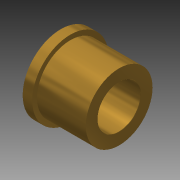
# Autodesk Inventor part: Ball Shisting Shaft Outline Sketch
Saved by Autodesk Inventor 2013 (Build 170138000, 138)
## iProperties
Created: 2013-06-04
Part Number: Ball Shisting Shaft Outline Sketch
Material: Generic
Document SubType Name: Modeling
Designer: mvarma
Density: 1 g/cm^3
Author: mvarma
Autodesk Inventor part; units mm, degrees
ref_plane "YZ Plane" through (0, 0, 0) normal (1, 0, 0) x (0, 1, 0)
ref_plane "XZ Plane" through (0, 0, 0) normal (0, 1, 0) x (-1, 0, 0)
ref_plane "XY Plane" through (0, 0, 0) normal (0, 0, 1) x (1, 0, 0)
sketch "Sketch1" plane through (0, 0, 0) normal (0, 0, 1) x (1, 0, 0)
  line L0 (0, 0) -> (0, 5.5563) construction
  line L1 (0, 0) -> (7.1437, 0) construction
  line L2 (7.1437, 0) -> (7.3977, 0) construction
  line L3 (0, 6.35) -> (7.1437, 6.35) construction
  line L4 (7.1437, 6.35) -> (7.1437, 0) construction
  line L5 (0, 5.5563) -> (7.1437, 5.5563)
  line L6 (7.1437, 6.35) -> (7.1437, 7.9375) construction
  line L7 (7.1437, 7.9375) -> (33.4328, 7.9375) construction
  line L8 (33.4328, 0) -> (33.4328, 7.9375) construction
  line L9 (33.4328, 7.3323) -> (36.6078, 7.3323) construction
  line L10 (36.6078, 7.3323) -> (36.6078, 0) construction
  line L11 (36.6078, 0) -> (33.4328, 0) construction
  line L12 (36.6078, 6.35) -> (44.0055, 6.35) construction
  line L13 (44.0055, 6.35) -> (44.0055, 0) construction
  line L14 (36.6078, 0) -> (36.8618, 0) construction
  line L15 (36.8618, 0) -> (44.0055, 0) construction
  line L16 (36.8618, 0) -> (36.8618, 6.35) construction
  line L17 (7.1437, 5.5563) -> (8.1153, 5.5563)
  line L18 (16.4059, 7.874) -> (17.6759, 7.874) construction
  line L19 (0, 3.1115) -> (44.0055, 3.1115) construction
  line L20 (0, 5.1753) -> (44.0055, 5.1753) construction
  line L21 (7.3977, 0) -> (7.3977, 7.9375) construction
  line L22 (7.3977, 0) -> (8.1915, 0) construction
  line L23 (8.1915, 0) -> (8.1915, 7.9375) construction
  line L24 (8.1915, 7.9375) -> (8.1915, 25.0214) construction
  line L25 (8.1915, 25.0214) -> (12.954, 25.0214) construction
  line L26 (12.954, 25.0214) -> (12.954, 0) construction
  line L27 (12.954, 0) -> (8.1915, 0) construction
  line L28 (12.954, 17.4625) -> (20.2882, 17.4625) construction
  line L29 (12.954, 25.0214) -> (17.7165, 25.0214) construction
  line L30 (17.7165, 25.0214) -> (17.7165, 0) construction
  line L31 (17.7165, 0) -> (12.954, 0) construction
  line L32 (20.2882, 17.4625) -> (20.2882, 0) construction
  line L33 (20.2882, 0) -> (17.7165, 0) construction
  line L34 (20.2882, 0) -> (21.082, 0) construction
  line L35 (21.082, 0) -> (21.082, 14.2875) construction
  line L36 (21.082, 14.2875) -> (20.2882, 14.2875) construction
  line L37 (7.3977, 7.9375) -> (7.3977, 14.2875) construction
  line L38 (7.3977, 14.2875) -> (8.1915, 14.2875) construction
  line L39 (21.082, 30.0415) -> (25.8445, 30.0415) construction
  line L40 (25.8445, 30.0415) -> (25.8445, 0) construction
  line L41 (25.8445, 0) -> (21.082, 0) construction
  line L42 (25.8445, 30.0415) -> (30.607, 30.0415) construction
  line L43 (30.607, 30.0415) -> (30.607, 0) construction
  line L44 (25.8445, 0) -> (30.607, 0) construction
  line L45 (25.8445, 17.4625) -> (33.1787, 17.4625) construction
  line L46 (33.1787, 17.4625) -> (33.1787, 0) construction
  line L47 (33.1787, 0) -> (30.607, 0) construction
  line L48 (21.082, 14.2875) -> (21.082, 30.0415) construction
  line L49 (33.1787, 0) -> (33.4328, 0) construction
  line L50 (10.5727, 25.0214) -> (10.5727, 0) construction
  line L51 (23.4632, 30.0415) -> (23.4632, 0) construction
  circle A0 centre (10.5727, 7.5565) radius 2.3813 construction
  circle A1 centre (10.5727, 5.4928) radius 2.3813 construction
  line L52 (8.9893, 7.874) -> (10.2593, 7.874) construction
  circle A2 centre (23.4632, 5.4928) radius 2.3812 construction
  circle A3 centre (23.4632, 7.5565) radius 2.3812 construction
  line L53 (23.0177, 7.874) -> (24.0459, 7.874) construction
  line L54 (13.843, 5.1752) -> (11.7793, 3.1115) construction
  line L55 (20.193, 5.1752) -> (22.2567, 3.1115) construction
  line L56 (9.9377, 5.1753) -> (7.874, 3.1115) construction
  line L57 (9.6837, 5.1752) -> (8.1153, 3.6068) construction
  line L58 (0, 3.5719) -> (8.0804, 3.5719)
  line L59 (0, 3.5719) -> (-1.5875, 3.5719)
  line L60 (-1.5875, 3.5719) -> (-1.5875, 6.35)
  line L61 (-1.5875, 6.35) -> (0, 6.35)
  line L62 (25.9207, 7.9375) -> (25.9207, 0) construction
  line L63 (24.0982, 5.1752) -> (26.162, 3.1115) construction
  line L64 (25.9207, 5.5563) -> (27.3897, 3.1115) construction
  line L65 (16.0338, 5.1752) -> (18.0975, 3.1115) construction
  line L66 (36.7242, 3.1115) -> (36.7242, 0) construction
  line L67 (15.6845, 3.1115) -> (17.7482, 5.1753) construction
  line L68 (69.3538, 20.0694) -> (73.1082, 25.272) construction
  line L69 (73.1082, 25.272) -> (79.491, 24.6219) construction
  line L70 (79.491, 24.6219) -> (82.1194, 18.7692) construction
  line L71 (82.1194, 18.7692) -> (78.365, 13.5666) construction
  line L72 (78.365, 13.5666) -> (71.9822, 14.2167) construction
  line L73 (71.9822, 14.2167) -> (69.3538, 20.0694) construction
  circle A4 centre (75.7366, 19.4193) radius 6.4158 construction
  line L74 (44.0055, 5.5563) -> (53.7803, 5.5563) construction
  line L75 (53.7803, 5.5563) -> (53.7803, 0) construction
  line L76 (53.7803, 0) -> (44.0055, 0) construction
  line L77 (27.2323, 3.3734) -> (44.0055, 3.3734) construction
  line L78 (30.5292, 0) -> (28.6597, 3.1115) construction
  line L79 (36.7242, 3.1115) -> (38.5937, 0) construction
  line L80 (36.9782, 3.1115) -> (38.8477, 0) construction
  line L81 (8.1153, 7.9375) -> (8.1153, 5.5563) construction
  line L82 (36.9782, 3.1115) -> (36.8208, 3.3734) construction
  line L83 (0, 5.5563) -> (0, 6.35)
  line L84 (8.1153, 3.6068) -> (8.0804, 3.5719)
  line L85 (8.0804, 3.5719) -> (7.62, 3.1115) construction
  line L86 (8.1153, 3.6068) -> (8.1153, 0) construction
  line L87 (8.1153, 5.5563) -> (8.1153, 3.6068)
  line L88 (8.1153, 5.5563) -> (44.0055, 5.5563) construction
  point P0 (10.5727, 3.1115)
  point P1 (10.5727, 5.1753)
  point P2 (23.4632, 5.1753)
  dimension "d78" = 4.7625
  dimension "d82" = 4.7625
  dimension "d116" = 12.8316
  dimension "d40" = 0.254
  dimension "d41" = 7.1437
  dimension "d42" = 6.35
  dimension "d43" = 5.5563
  dimension "d44" = 7.9375
  dimension "d46" = 7.3323
  dimension "d47" = 3.175
  dimension "d48" = 0.254
  dimension "d49" = 6.35
  dimension "d50" = 7.1437
  dimension "d53" = 1.27
  dimension "d54" = 0.0635
  dimension "d58" = 3.1115
  dimension "d61" = 5.1753
  dimension "d63" = 0.7937
  dimension "d64" = 4.7625
  dimension "d65" = 7.3342
  dimension "d66" = 17.4625
  dimension "d67" = 4.7625
  dimension "d68" = 0.7937
  dimension "d69" = 14.2875
  dimension "d70" = 14.2875
  dimension "d71" = 4.7625
  dimension "d72" = 4.7625
  dimension "d73" = 7.3342
  dimension "d74" = 17.4625
  dimension "d75" = 0.254
  dimension "d76" = 12.8905
  dimension "d77" = 0.381
  dimension "d80" = 0.0635
  dimension "d81" = 4.7625
  dimension "d83" = 0.381
  dimension "d84" = 0.0635
  dimension "d85" = 45
  dimension "d86" = 45
  dimension "d88" = 1.2065
  dimension "d89" = 6.35
  dimension "d90" = 3.2702
  dimension "d91" = 0.635
  dimension "d92" = 45
  dimension "d93" = 0.254
  dimension "d94" = 3.5719
  dimension "d95" = 0.4604
  dimension "d96" = 1.5875
  dimension "d97" = 2.7781
  dimension "d98" = 1.6034
  dimension "d99" = 3.9053
  dimension "d101" = 3.2702
  dimension "d102" = 4.9149
  dimension "d103" = 0.635
  dimension "d105" = 59
  dimension "d106" = 2.4977
  dimension "d107" = 6.35
  dimension "d108" = 45
  dimension "d109" = 8.0645
  dimension "d110" = 10.5622
  dimension "d114" = 6.35
  dimension "d115" = 11.1125
  dimension "d117" = 5.5563
  dimension "d118" = 3.1115
  dimension "d120" = 3.3734
  dimension "d121" = 59
  dimension "d122" = 1.27
  dimension "d123" = 59
  constraints: 174 end point, 44 perpendicular, 40 point on line, 18 parallel, 7 collinear, 5 horizontal, 5 vertical, 4 midpoint, 3 vertical alignment, 1 centre point, 1 coincident, 1 tangent, 46 other
  measures "d40" distance of L1.end L2.end
  measures "d41" distance of L0.start L1.end
  measures "d42" distance between parallel lines of L1 L3
  measures "d43" distance between parallel lines of L1 L5
  measures "d44" distance from line of L0.start L7
  measures "d46" distance from line of L8.start L9
  measures "d47" distance of L9.start L9.end
  measures "d48" distance of L10.end L14.end
  measures "d49" distance between parallel lines of L15 L12
  measures "d50" distance of L14.end L13.end
  measures "d53" distance of L18.start L18.end
  measures "d54" distance between parallel lines of L7 L18
  measures "d63" distance of L2.end L22.end
  measures "d64" distance of L24.end L25.end
  measures "d65" distance of L28.start L28.end
  measures "d66" distance between parallel lines of L27 L28
  measures "d67" distance of L25.end L29.end
  measures "d68" distance of L32.end L34.end
  measures "d69" distance between parallel lines of L34 L36
  measures "d70" distance between parallel lines of L22 L38
  measures "d71" distance of L39.start L39.end
  measures "d72" distance of L39.end L42.end
  measures "d73" distance of L45.start L45.end
  measures "d74" distance between parallel lines of L44 L45
  measures "d75" distance of L46.end L8.start
  measures "d76" distance between parallel lines of L51 L50
  measures "d77" distance from line of L7 point (10.573, 7.557)
  measures "d80" distance between parallel lines of L7 L52
  measures "d81" diameter of A2
  measures "d83" distance from line of L7 point (23.463, 7.557)
  measures "d84" distance between parallel lines of L7 L53
  measures "d85" angle to the sketch x axis of L54
  measures "d86" angle to the sketch x axis of L55
  measures "d88" distance of point (10.573, 3.112) L54.end
  measures "d89" distance of L55.start L54.start
  measures "d90" distance of L54.start point (10.573, 5.175)
  measures "d91" distance of point (10.573, 5.175) L56.start
  measures "d92" angle to the sketch x axis of L56
  measures "d93" distance of L56.start L57.start
  measures "d94" distance between parallel lines of L1 L58
  measures "d96" distance between parallel lines of L0 L60
  measures "d97" distance between parallel lines of L3 L58
  measures "d99" distance of L54.start L56.start
  measures "d101" distance of point (23.463, 5.175) L55.start
  measures "d102" diameter of L62 L51
  measures "d103" distance of point (23.463, 5.175) L63.start
  measures "d105" angle to the sketch x axis of L64
  measures "d106" distance of L78.end L63.end
  measures "d107" distance of L65.start L57.start
  measures "d108" angle to the sketch x axis of L65
  measures "d109" distance of L63.start L65.start
  measures "d110" distance of L66.start L63.end
  measures "d114" distance of L63.start L67.end
  measures "d115" distance between parallel lines of L72 L69
  measures "d117" distance between parallel lines of L76 L74
  measures "d120" distance between parallel lines of L47 L77
  measures "d121" angle of L44 L78
  measures "d122" distance of L64.end L78.end
  measures "d123" angle of L15 L79
revolve "Revolution1" add sketch "Sketch1" angle 360 about axis through (20.2882, 0, 0) along (-1, 0, 0)
body "Solid1"
